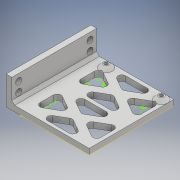
# Autodesk Inventor part: OpenMV
Saved by Autodesk Inventor 2018 (Build 220112000, 112)
## iProperties
Created: 2018-09-23
Part Number: OpenMV
Material: 一般
Document SubType Name: Modeling
Designer: shun2
Density: 1 g/cm^3
Appearance: 既定
Author: shun2
Autodesk Inventor part; units mm, degrees
ref_plane "YZ Plane" through (0, 0, 0) normal (1, 0, 0) x (0, 1, 0)
ref_plane "XZ Plane" through (0, 0, 0) normal (0, 1, 0) x (-1, 0, 0)
ref_plane "XY Plane" through (0, 0, 0) normal (0, 0, 1) x (1, 0, 0)
sketch "スケッチ2" plane through (0, 0, 0) normal (0, 0, 1) x (1, 0, 0)
  line L0 (0, 44.45) -> (0, 0)
  line L1 (0, 0) -> (35.56, 0)
  line L2 (35.56, 0) -> (35.56, 44.45)
  line L3 (35.56, 44.45) -> (0, 44.45)
  arc A0 (0.381, 41.1607) -> (0.381, 41.1353) centre (0.381, 41.148) ccw
  arc A1 (6.223, 41.1353) -> (6.223, 41.1607) centre (6.223, 41.148) ccw
  arc A2 (3.302, 38.227) -> (3.302, 44.069) centre (3.302, 41.148) ccw
  arc A3 (3.302, 44.069) -> (3.302, 38.227) centre (3.302, 41.148) ccw
  arc A4 (3.302, 39.648) -> (3.302, 42.648) centre (3.302, 41.148) ccw
  arc A5 (3.302, 42.648) -> (3.302, 39.648) centre (3.302, 41.148) ccw
  line L4 (35.179, 41.148) -> (34.925, 41.148)
  arc A6 (34.925, 41.1607) -> (34.925, 41.1353) centre (34.925, 41.148) ccw
  arc A7 (35.179, 41.1353) -> (35.179, 41.1607) centre (35.179, 41.148) ccw
  arc A8 (29.337, 41.1607) -> (29.337, 41.1353) centre (29.337, 41.148) ccw
  arc A9 (32.258, 38.227) -> (32.258, 44.069) centre (32.258, 41.148) ccw
  arc A10 (32.258, 44.069) -> (32.258, 38.227) centre (32.258, 41.148) ccw
  arc A11 (32.258, 39.648) -> (32.258, 42.648) centre (32.258, 41.148) ccw
  arc A12 (32.258, 42.648) -> (32.258, 39.648) centre (32.258, 41.148) ccw
  line L5 (35.179, 4.699) -> (35.179, 3.429)
  arc A13 (35.1409, 3.429) -> (35.2171, 3.429) centre (35.179, 3.429) ccw
  arc A14 (35.2171, 4.699) -> (35.1409, 4.699) centre (35.179, 4.699) ccw
  line L6 (35.179, 3.429) -> (34.544, 2.794)
  arc A15 (34.5171, 2.8209) -> (34.5709, 2.7671) centre (34.544, 2.794) ccw
  arc A16 (35.2059, 3.4021) -> (35.1521, 3.4559) centre (35.179, 3.429) ccw
  arc A17 (33.274, 2.8321) -> (33.274, 2.7559) centre (33.274, 2.794) ccw
  arc A18 (34.544, 2.7559) -> (34.544, 2.8321) centre (34.544, 2.794) ccw
  line L7 (33.274, 2.794) -> (32.639, 3.429)
  arc A19 (32.6659, 3.4559) -> (32.6121, 3.4021) centre (32.639, 3.429) ccw
  arc A20 (33.2471, 2.7671) -> (33.3009, 2.8209) centre (33.274, 2.794) ccw
  line L8 (34.544, 7.874) -> (35.179, 7.239)
  arc A21 (35.1521, 7.2121) -> (35.2059, 7.2659) centre (35.179, 7.239) ccw
  arc A22 (34.5709, 7.9009) -> (34.5171, 7.8471) centre (34.544, 7.874) ccw
  line L9 (35.179, 7.239) -> (35.179, 5.969)
  arc A23 (35.1409, 5.969) -> (35.2171, 5.969) centre (35.179, 5.969) ccw
  arc A24 (35.2171, 7.239) -> (35.1409, 7.239) centre (35.179, 7.239) ccw
  line L10 (35.179, 5.969) -> (34.544, 5.334)
  arc A25 (34.5171, 5.3609) -> (34.5709, 5.3071) centre (34.544, 5.334) ccw
  arc A26 (35.2059, 5.9421) -> (35.1521, 5.9959) centre (35.179, 5.969) ccw
  arc A27 (33.274, 5.3721) -> (33.274, 5.2959) centre (33.274, 5.334) ccw
  arc A28 (34.544, 5.2959) -> (34.544, 5.3721) centre (34.544, 5.334) ccw
  line L11 (33.274, 5.334) -> (32.639, 5.969)
  arc A29 (32.6659, 5.9959) -> (32.6121, 5.9421) centre (32.639, 5.969) ccw
  arc A30 (33.2471, 5.3071) -> (33.3009, 5.3609) centre (33.274, 5.334) ccw
  line L12 (32.639, 5.969) -> (32.639, 7.239)
  arc A31 (32.6771, 7.239) -> (32.6009, 7.239) centre (32.639, 7.239) ccw
  arc A32 (32.6009, 5.969) -> (32.6771, 5.969) centre (32.639, 5.969) ccw
  line L13 (32.639, 7.239) -> (33.274, 7.874)
  arc A33 (33.3009, 7.8471) -> (33.2471, 7.9009) centre (33.274, 7.874) ccw
  arc A34 (32.6121, 7.2659) -> (32.6659, 7.2121) centre (32.639, 7.239) ccw
  line L14 (35.179, 4.699) -> (34.544, 5.334)
  arc A35 (34.5709, 5.3609) -> (34.5171, 5.3071) centre (34.544, 5.334) ccw
  arc A36 (35.1521, 4.6721) -> (35.2059, 4.7259) centre (35.179, 4.699) ccw
  line L15 (33.274, 5.334) -> (32.639, 4.699)
  arc A37 (32.6121, 4.7259) -> (32.6659, 4.6721) centre (32.639, 4.699) ccw
  arc A38 (33.3009, 5.3071) -> (33.2471, 5.3609) centre (33.274, 5.334) ccw
  line L16 (32.639, 3.429) -> (32.639, 4.699)
  arc A39 (32.6771, 4.699) -> (32.6009, 4.699) centre (32.639, 4.699) ccw
  arc A40 (32.6009, 3.429) -> (32.6771, 3.429) centre (32.639, 3.429) ccw
  line L17 (35.179, 12.319) -> (35.179, 11.049)
  arc A41 (35.1409, 11.049) -> (35.2171, 11.049) centre (35.179, 11.049) ccw
  arc A42 (35.2171, 12.319) -> (35.1409, 12.319) centre (35.179, 12.319) ccw
  line L18 (35.179, 11.049) -> (34.544, 10.414)
  arc A43 (34.5171, 10.4409) -> (34.5709, 10.3871) centre (34.544, 10.414) ccw
  arc A44 (35.2059, 11.0221) -> (35.1521, 11.0759) centre (35.179, 11.049) ccw
  arc A45 (33.274, 10.4521) -> (33.274, 10.3759) centre (33.274, 10.414) ccw
  arc A46 (34.544, 10.3759) -> (34.544, 10.4521) centre (34.544, 10.414) ccw
  line L19 (33.274, 10.414) -> (32.639, 11.049)
  arc A47 (32.6659, 11.0759) -> (32.6121, 11.0221) centre (32.639, 11.049) ccw
  arc A48 (33.2471, 10.3871) -> (33.3009, 10.4409) centre (33.274, 10.414) ccw
  line L20 (34.544, 10.414) -> (35.179, 9.779)
  arc A49 (35.1521, 9.7521) -> (35.2059, 9.8059) centre (35.179, 9.779) ccw
  arc A50 (34.5709, 10.4409) -> (34.5171, 10.3871) centre (34.544, 10.414) ccw
  line L21 (35.179, 9.779) -> (35.179, 8.509)
  arc A51 (35.1409, 8.509) -> (35.2171, 8.509) centre (35.179, 8.509) ccw
  arc A52 (35.2171, 9.779) -> (35.1409, 9.779) centre (35.179, 9.779) ccw
  line L22 (35.179, 8.509) -> (34.544, 7.874)
  arc A53 (34.5171, 7.9009) -> (34.5709, 7.8471) centre (34.544, 7.874) ccw
  arc A54 (35.2059, 8.4821) -> (35.1521, 8.5359) centre (35.179, 8.509) ccw
  arc A55 (33.274, 7.9121) -> (33.274, 7.8359) centre (33.274, 7.874) ccw
  arc A56 (34.544, 7.8359) -> (34.544, 7.9121) centre (34.544, 7.874) ccw
  line L23 (33.274, 7.874) -> (32.639, 8.509)
  arc A57 (32.6659, 8.5359) -> (32.6121, 8.4821) centre (32.639, 8.509) ccw
  arc A58 (33.2471, 7.8471) -> (33.3009, 7.9009) centre (33.274, 7.874) ccw
  line L24 (32.639, 8.509) -> (32.639, 9.779)
  arc A59 (32.6771, 9.779) -> (32.6009, 9.779) centre (32.639, 9.779) ccw
  arc A60 (32.6009, 8.509) -> (32.6771, 8.509) centre (32.639, 8.509) ccw
  line L25 (32.639, 9.779) -> (33.274, 10.414)
  arc A61 (33.3009, 10.3871) -> (33.2471, 10.4409) centre (33.274, 10.414) ccw
  arc A62 (32.6121, 9.8059) -> (32.6659, 9.7521) centre (32.639, 9.779) ccw
  line L26 (34.544, 15.494) -> (35.179, 14.859)
  arc A63 (35.1521, 14.8321) -> (35.2059, 14.8859) centre (35.179, 14.859) ccw
  arc A64 (34.5709, 15.5209) -> (34.5171, 15.4671) centre (34.544, 15.494) ccw
  line L27 (35.179, 14.859) -> (35.179, 13.589)
  arc A65 (35.1409, 13.589) -> (35.2171, 13.589) centre (35.179, 13.589) ccw
  arc A66 (35.2171, 14.859) -> (35.1409, 14.859) centre (35.179, 14.859) ccw
  line L28 (35.179, 13.589) -> (34.544, 12.954)
  arc A67 (34.5171, 12.9809) -> (34.5709, 12.9271) centre (34.544, 12.954) ccw
  arc A68 (35.2059, 13.5621) -> (35.1521, 13.6159) centre (35.179, 13.589) ccw
  arc A69 (33.274, 12.9921) -> (33.274, 12.9159) centre (33.274, 12.954) ccw
  arc A70 (34.544, 12.9159) -> (34.544, 12.9921) centre (34.544, 12.954) ccw
  line L29 (33.274, 12.954) -> (32.639, 13.589)
  arc A71 (32.6659, 13.6159) -> (32.6121, 13.5621) centre (32.639, 13.589) ccw
  arc A72 (33.2471, 12.9271) -> (33.3009, 12.9809) centre (33.274, 12.954) ccw
  line L30 (32.639, 13.589) -> (32.639, 14.859)
  arc A73 (32.6771, 14.859) -> (32.6009, 14.859) centre (32.639, 14.859) ccw
  arc A74 (32.6009, 13.589) -> (32.6771, 13.589) centre (32.639, 13.589) ccw
  line L31 (32.639, 14.859) -> (33.274, 15.494)
  arc A75 (33.3009, 15.4671) -> (33.2471, 15.5209) centre (33.274, 15.494) ccw
  arc A76 (32.6121, 14.8859) -> (32.6659, 14.8321) centre (32.639, 14.859) ccw
  line L32 (35.179, 12.319) -> (34.544, 12.954)
  arc A77 (34.5709, 12.9809) -> (34.5171, 12.9271) centre (34.544, 12.954) ccw
  arc A78 (35.1521, 12.2921) -> (35.2059, 12.3459) centre (35.179, 12.319) ccw
  line L33 (33.274, 12.954) -> (32.639, 12.319)
  arc A79 (32.6121, 12.3459) -> (32.6659, 12.2921) centre (32.639, 12.319) ccw
  arc A80 (33.3009, 12.9271) -> (33.2471, 12.9809) centre (33.274, 12.954) ccw
  line L34 (32.639, 11.049) -> (32.639, 12.319)
  arc A81 (32.6771, 12.319) -> (32.6009, 12.319) centre (32.639, 12.319) ccw
  arc A82 (32.6009, 11.049) -> (32.6771, 11.049) centre (32.639, 11.049) ccw
  line L35 (35.179, 19.939) -> (35.179, 18.669)
  arc A83 (35.1409, 18.669) -> (35.2171, 18.669) centre (35.179, 18.669) ccw
  arc A84 (35.2171, 19.939) -> (35.1409, 19.939) centre (35.179, 19.939) ccw
  line L36 (35.179, 18.669) -> (34.544, 18.034)
  arc A85 (34.5171, 18.0609) -> (34.5709, 18.0071) centre (34.544, 18.034) ccw
  arc A86 (35.2059, 18.6421) -> (35.1521, 18.6959) centre (35.179, 18.669) ccw
  arc A87 (33.274, 18.0721) -> (33.274, 17.9959) centre (33.274, 18.034) ccw
  arc A88 (34.544, 17.9959) -> (34.544, 18.0721) centre (34.544, 18.034) ccw
  line L37 (33.274, 18.034) -> (32.639, 18.669)
  arc A89 (32.6659, 18.6959) -> (32.6121, 18.6421) centre (32.639, 18.669) ccw
  arc A90 (33.2471, 18.0071) -> (33.3009, 18.0609) centre (33.274, 18.034) ccw
  line L38 (34.544, 18.034) -> (35.179, 17.399)
  arc A91 (35.1521, 17.3721) -> (35.2059, 17.4259) centre (35.179, 17.399) ccw
  arc A92 (34.5709, 18.0609) -> (34.5171, 18.0071) centre (34.544, 18.034) ccw
  line L39 (35.179, 17.399) -> (35.179, 16.129)
  arc A93 (35.1409, 16.129) -> (35.2171, 16.129) centre (35.179, 16.129) ccw
  arc A94 (35.2171, 17.399) -> (35.1409, 17.399) centre (35.179, 17.399) ccw
  line L40 (35.179, 16.129) -> (34.544, 15.494)
  arc A95 (34.5171, 15.5209) -> (34.5709, 15.4671) centre (34.544, 15.494) ccw
  arc A96 (35.2059, 16.1021) -> (35.1521, 16.1559) centre (35.179, 16.129) ccw
  arc A97 (33.274, 15.5321) -> (33.274, 15.4559) centre (33.274, 15.494) ccw
  arc A98 (34.544, 15.4559) -> (34.544, 15.5321) centre (34.544, 15.494) ccw
  line L41 (33.274, 15.494) -> (32.639, 16.129)
  arc A99 (32.6659, 16.1559) -> (32.6121, 16.1021) centre (32.639, 16.129) ccw
  arc A100 (33.2471, 15.4671) -> (33.3009, 15.5209) centre (33.274, 15.494) ccw
  line L42 (32.639, 16.129) -> (32.639, 17.399)
  arc A101 (32.6771, 17.399) -> (32.6009, 17.399) centre (32.639, 17.399) ccw
  arc A102 (32.6009, 16.129) -> (32.6771, 16.129) centre (32.639, 16.129) ccw
  line L43 (32.639, 17.399) -> (33.274, 18.034)
  arc A103 (33.3009, 18.0071) -> (33.2471, 18.0609) centre (33.274, 18.034) ccw
  arc A104 (32.6121, 17.4259) -> (32.6659, 17.3721) centre (32.639, 17.399) ccw
  line L44 (34.544, 20.574) -> (33.274, 20.574)
  arc A105 (33.274, 20.6121) -> (33.274, 20.5359) centre (33.274, 20.574) ccw
  arc A106 (34.544, 20.5359) -> (34.544, 20.6121) centre (34.544, 20.574) ccw
  line L45 (35.179, 19.939) -> (34.544, 20.574)
  arc A107 (34.5709, 20.6009) -> (34.5171, 20.5471) centre (34.544, 20.574) ccw
  arc A108 (35.1521, 19.9121) -> (35.2059, 19.9659) centre (35.179, 19.939) ccw
  line L46 (33.274, 20.574) -> (32.639, 19.939)
  arc A109 (32.6121, 19.9659) -> (32.6659, 19.9121) centre (32.639, 19.939) ccw
  arc A110 (33.3009, 20.5471) -> (33.2471, 20.6009) centre (33.274, 20.574) ccw
  line L47 (32.639, 18.669) -> (32.639, 19.939)
  arc A111 (32.6771, 19.939) -> (32.6009, 19.939) centre (32.639, 19.939) ccw
  arc A112 (32.6009, 18.669) -> (32.6771, 18.669) centre (32.639, 18.669) ccw
  line L48 (35.179, 2.159) -> (35.179, 0.889)
  arc A113 (35.1409, 0.889) -> (35.2171, 0.889) centre (35.179, 0.889) ccw
  arc A114 (35.2171, 2.159) -> (35.1409, 2.159) centre (35.179, 2.159) ccw
  line L49 (35.179, 0.889) -> (34.544, 0.254)
  arc A115 (34.5171, 0.2809) -> (34.5709, 0.2271) centre (34.544, 0.254) ccw
  arc A116 (35.2059, 0.8621) -> (35.1521, 0.9159) centre (35.179, 0.889) ccw
  line L50 (34.544, 0.254) -> (33.274, 0.254)
  arc A117 (33.274, 0.2921) -> (33.274, 0.2159) centre (33.274, 0.254) ccw
  arc A118 (34.544, 0.2159) -> (34.544, 0.2921) centre (34.544, 0.254) ccw
  line L51 (33.274, 0.254) -> (32.639, 0.889)
  arc A119 (32.6659, 0.9159) -> (32.6121, 0.8621) centre (32.639, 0.889) ccw
  arc A120 (33.2471, 0.2271) -> (33.3009, 0.2809) centre (33.274, 0.254) ccw
  line L52 (35.179, 2.159) -> (34.544, 2.794)
  arc A121 (34.5709, 2.8209) -> (34.5171, 2.7671) centre (34.544, 2.794) ccw
  arc A122 (35.1521, 2.1321) -> (35.2059, 2.1859) centre (35.179, 2.159) ccw
  line L53 (33.274, 2.794) -> (32.639, 2.159)
  arc A123 (32.6121, 2.1859) -> (32.6659, 2.1321) centre (32.639, 2.159) ccw
  arc A124 (33.3009, 2.7671) -> (33.2471, 2.8209) centre (33.274, 2.794) ccw
  line L54 (32.639, 0.889) -> (32.639, 2.159)
  arc A125 (32.6771, 2.159) -> (32.6009, 2.159) centre (32.639, 2.159) ccw
  arc A126 (32.6009, 0.889) -> (32.6771, 0.889) centre (32.639, 0.889) ccw
  line L55 (2.921, 4.699) -> (2.921, 3.429)
  arc A127 (2.8829, 3.429) -> (2.9591, 3.429) centre (2.921, 3.429) ccw
  arc A128 (2.9591, 4.699) -> (2.8829, 4.699) centre (2.921, 4.699) ccw
  line L56 (2.921, 3.429) -> (2.286, 2.794)
  arc A129 (2.2591, 2.8209) -> (2.3129, 2.7671) centre (2.286, 2.794) ccw
  arc A130 (2.9479, 3.4021) -> (2.8941, 3.4559) centre (2.921, 3.429) ccw
  arc A131 (1.016, 2.8321) -> (1.016, 2.7559) centre (1.016, 2.794) ccw
  arc A132 (2.286, 2.7559) -> (2.286, 2.8321) centre (2.286, 2.794) ccw
  line L57 (1.016, 2.794) -> (0.381, 3.429)
  arc A133 (0.4079, 3.4559) -> (0.3541, 3.4021) centre (0.381, 3.429) ccw
  arc A134 (0.9891, 2.7671) -> (1.0429, 2.8209) centre (1.016, 2.794) ccw
  line L58 (2.286, 7.874) -> (2.921, 7.239)
  arc A135 (2.8941, 7.2121) -> (2.9479, 7.2659) centre (2.921, 7.239) ccw
  arc A136 (2.3129, 7.9009) -> (2.2591, 7.8471) centre (2.286, 7.874) ccw
  line L59 (2.921, 7.239) -> (2.921, 5.969)
  arc A137 (2.8829, 5.969) -> (2.9591, 5.969) centre (2.921, 5.969) ccw
  arc A138 (2.9591, 7.239) -> (2.8829, 7.239) centre (2.921, 7.239) ccw
  line L60 (2.921, 5.969) -> (2.286, 5.334)
  arc A139 (2.2591, 5.3609) -> (2.3129, 5.3071) centre (2.286, 5.334) ccw
  arc A140 (2.9479, 5.9421) -> (2.8941, 5.9959) centre (2.921, 5.969) ccw
  arc A141 (1.016, 5.3721) -> (1.016, 5.2959) centre (1.016, 5.334) ccw
  arc A142 (2.286, 5.2959) -> (2.286, 5.3721) centre (2.286, 5.334) ccw
  line L61 (1.016, 5.334) -> (0.381, 5.969)
  arc A143 (0.4079, 5.9959) -> (0.3541, 5.9421) centre (0.381, 5.969) ccw
  arc A144 (0.9891, 5.3071) -> (1.0429, 5.3609) centre (1.016, 5.334) ccw
  line L62 (0.381, 5.969) -> (0.381, 7.239)
  arc A145 (0.4191, 7.239) -> (0.3429, 7.239) centre (0.381, 7.239) ccw
  arc A146 (0.3429, 5.969) -> (0.4191, 5.969) centre (0.381, 5.969) ccw
  line L63 (0.381, 7.239) -> (1.016, 7.874)
  arc A147 (1.0429, 7.8471) -> (0.9891, 7.9009) centre (1.016, 7.874) ccw
  arc A148 (0.3541, 7.2659) -> (0.4079, 7.2121) centre (0.381, 7.239) ccw
  line L64 (2.921, 4.699) -> (2.286, 5.334)
  arc A149 (2.3129, 5.3609) -> (2.2591, 5.3071) centre (2.286, 5.334) ccw
  arc A150 (2.8941, 4.6721) -> (2.9479, 4.7259) centre (2.921, 4.699) ccw
  line L65 (1.016, 5.334) -> (0.381, 4.699)
  arc A151 (0.3541, 4.7259) -> (0.4079, 4.6721) centre (0.381, 4.699) ccw
  arc A152 (1.0429, 5.3071) -> (0.9891, 5.3609) centre (1.016, 5.334) ccw
  line L66 (0.381, 3.429) -> (0.381, 4.699)
  arc A153 (0.4191, 4.699) -> (0.3429, 4.699) centre (0.381, 4.699) ccw
  arc A154 (0.3429, 3.429) -> (0.4191, 3.429) centre (0.381, 3.429) ccw
  line L67 (2.921, 12.319) -> (2.921, 11.049)
  arc A155 (2.8829, 11.049) -> (2.9591, 11.049) centre (2.921, 11.049) ccw
  arc A156 (2.9591, 12.319) -> (2.8829, 12.319) centre (2.921, 12.319) ccw
  line L68 (2.921, 11.049) -> (2.286, 10.414)
  arc A157 (2.2591, 10.4409) -> (2.3129, 10.3871) centre (2.286, 10.414) ccw
  arc A158 (2.9479, 11.0221) -> (2.8941, 11.0759) centre (2.921, 11.049) ccw
  arc A159 (1.016, 10.4521) -> (1.016, 10.3759) centre (1.016, 10.414) ccw
  arc A160 (2.286, 10.3759) -> (2.286, 10.4521) centre (2.286, 10.414) ccw
  line L69 (1.016, 10.414) -> (0.381, 11.049)
  arc A161 (0.4079, 11.0759) -> (0.3541, 11.0221) centre (0.381, 11.049) ccw
  arc A162 (0.9891, 10.3871) -> (1.0429, 10.4409) centre (1.016, 10.414) ccw
  line L70 (2.286, 10.414) -> (2.921, 9.779)
  arc A163 (2.8941, 9.7521) -> (2.9479, 9.8059) centre (2.921, 9.779) ccw
  arc A164 (2.3129, 10.4409) -> (2.2591, 10.3871) centre (2.286, 10.414) ccw
  line L71 (2.921, 9.779) -> (2.921, 8.509)
  arc A165 (2.8829, 8.509) -> (2.9591, 8.509) centre (2.921, 8.509) ccw
  arc A166 (2.9591, 9.779) -> (2.8829, 9.779) centre (2.921, 9.779) ccw
  line L72 (2.921, 8.509) -> (2.286, 7.874)
  arc A167 (2.2591, 7.9009) -> (2.3129, 7.8471) centre (2.286, 7.874) ccw
  arc A168 (2.9479, 8.4821) -> (2.8941, 8.5359) centre (2.921, 8.509) ccw
  arc A169 (1.016, 7.9121) -> (1.016, 7.8359) centre (1.016, 7.874) ccw
  arc A170 (2.286, 7.8359) -> (2.286, 7.9121) centre (2.286, 7.874) ccw
  line L73 (1.016, 7.874) -> (0.381, 8.509)
  arc A171 (0.4079, 8.5359) -> (0.3541, 8.4821) centre (0.381, 8.509) ccw
  arc A172 (0.9891, 7.8471) -> (1.0429, 7.9009) centre (1.016, 7.874) ccw
  line L74 (0.381, 8.509) -> (0.381, 9.779)
  arc A173 (0.4191, 9.779) -> (0.3429, 9.779) centre (0.381, 9.779) ccw
  arc A174 (0.3429, 8.509) -> (0.4191, 8.509) centre (0.381, 8.509) ccw
  line L75 (0.381, 9.779) -> (1.016, 10.414)
  arc A175 (1.0429, 10.3871) -> (0.9891, 10.4409) centre (1.016, 10.414) ccw
  arc A176 (0.3541, 9.8059) -> (0.4079, 9.7521) centre (0.381, 9.779) ccw
  line L76 (2.286, 15.494) -> (2.921, 14.859)
  arc A177 (2.8941, 14.8321) -> (2.9479, 14.8859) centre (2.921, 14.859) ccw
  arc A178 (2.3129, 15.5209) -> (2.2591, 15.4671) centre (2.286, 15.494) ccw
  line L77 (2.921, 14.859) -> (2.921, 13.589)
  arc A179 (2.8829, 13.589) -> (2.9591, 13.589) centre (2.921, 13.589) ccw
  arc A180 (2.9591, 14.859) -> (2.8829, 14.859) centre (2.921, 14.859) ccw
  line L78 (2.921, 13.589) -> (2.286, 12.954)
  arc A181 (2.2591, 12.9809) -> (2.3129, 12.9271) centre (2.286, 12.954) ccw
  arc A182 (2.9479, 13.5621) -> (2.8941, 13.6159) centre (2.921, 13.589) ccw
  arc A183 (1.016, 12.9921) -> (1.016, 12.9159) centre (1.016, 12.954) ccw
  arc A184 (2.286, 12.9159) -> (2.286, 12.9921) centre (2.286, 12.954) ccw
  line L79 (1.016, 12.954) -> (0.381, 13.589)
  arc A185 (0.4079, 13.6159) -> (0.3541, 13.5621) centre (0.381, 13.589) ccw
  arc A186 (0.9891, 12.9271) -> (1.0429, 12.9809) centre (1.016, 12.954) ccw
  line L80 (0.381, 13.589) -> (0.381, 14.859)
  arc A187 (0.4191, 14.859) -> (0.3429, 14.859) centre (0.381, 14.859) ccw
  arc A188 (0.3429, 13.589) -> (0.4191, 13.589) centre (0.381, 13.589) ccw
  line L81 (0.381, 14.859) -> (1.016, 15.494)
  arc A189 (1.0429, 15.4671) -> (0.9891, 15.5209) centre (1.016, 15.494) ccw
  arc A190 (0.3541, 14.8859) -> (0.4079, 14.8321) centre (0.381, 14.859) ccw
  line L82 (2.921, 12.319) -> (2.286, 12.954)
  arc A191 (2.3129, 12.9809) -> (2.2591, 12.9271) centre (2.286, 12.954) ccw
  arc A192 (2.8941, 12.2921) -> (2.9479, 12.3459) centre (2.921, 12.319) ccw
  line L83 (1.016, 12.954) -> (0.381, 12.319)
  arc A193 (0.3541, 12.3459) -> (0.4079, 12.2921) centre (0.381, 12.319) ccw
  arc A194 (1.0429, 12.9271) -> (0.9891, 12.9809) centre (1.016, 12.954) ccw
  line L84 (0.381, 11.049) -> (0.381, 12.319)
  arc A195 (0.4191, 12.319) -> (0.3429, 12.319) centre (0.381, 12.319) ccw
  arc A196 (0.3429, 11.049) -> (0.4191, 11.049) centre (0.381, 11.049) ccw
  line L85 (2.921, 19.939) -> (2.921, 18.669)
  arc A197 (2.8829, 18.669) -> (2.9591, 18.669) centre (2.921, 18.669) ccw
  arc A198 (2.9591, 19.939) -> (2.8829, 19.939) centre (2.921, 19.939) ccw
  line L86 (2.921, 18.669) -> (2.286, 18.034)
  arc A199 (2.2591, 18.0609) -> (2.3129, 18.0071) centre (2.286, 18.034) ccw
  arc A200 (2.9479, 18.6421) -> (2.8941, 18.6959) centre (2.921, 18.669) ccw
  arc A201 (1.016, 18.0721) -> (1.016, 17.9959) centre (1.016, 18.034) ccw
  arc A202 (2.286, 17.9959) -> (2.286, 18.0721) centre (2.286, 18.034) ccw
  line L87 (1.016, 18.034) -> (0.381, 18.669)
  arc A203 (0.4079, 18.6959) -> (0.3541, 18.6421) centre (0.381, 18.669) ccw
  arc A204 (0.9891, 18.0071) -> (1.0429, 18.0609) centre (1.016, 18.034) ccw
  line L88 (2.286, 18.034) -> (2.921, 17.399)
  arc A205 (2.8941, 17.3721) -> (2.9479, 17.4259) centre (2.921, 17.399) ccw
  arc A206 (2.3129, 18.0609) -> (2.2591, 18.0071) centre (2.286, 18.034) ccw
  line L89 (2.921, 17.399) -> (2.921, 16.129)
  arc A207 (2.8829, 16.129) -> (2.9591, 16.129) centre (2.921, 16.129) ccw
  arc A208 (2.9591, 17.399) -> (2.8829, 17.399) centre (2.921, 17.399) ccw
  line L90 (2.921, 16.129) -> (2.286, 15.494)
  arc A209 (2.2591, 15.5209) -> (2.3129, 15.4671) centre (2.286, 15.494) ccw
  arc A210 (2.9479, 16.1021) -> (2.8941, 16.1559) centre (2.921, 16.129) ccw
  arc A211 (1.016, 15.5321) -> (1.016, 15.4559) centre (1.016, 15.494) ccw
  arc A212 (2.286, 15.4559) -> (2.286, 15.5321) centre (2.286, 15.494) ccw
  line L91 (1.016, 15.494) -> (0.381, 16.129)
  arc A213 (0.4079, 16.1559) -> (0.3541, 16.1021) centre (0.381, 16.129) ccw
  arc A214 (0.9891, 15.4671) -> (1.0429, 15.5209) centre (1.016, 15.494) ccw
  line L92 (0.381, 16.129) -> (0.381, 17.399)
  arc A215 (0.4191, 17.399) -> (0.3429, 17.399) centre (0.381, 17.399) ccw
  arc A216 (0.3429, 16.129) -> (0.4191, 16.129) centre (0.381, 16.129) ccw
  line L93 (0.381, 17.399) -> (1.016, 18.034)
  arc A217 (1.0429, 18.0071) -> (0.9891, 18.0609) centre (1.016, 18.034) ccw
  arc A218 (0.3541, 17.4259) -> (0.4079, 17.3721) centre (0.381, 17.399) ccw
  line L94 (2.286, 20.574) -> (1.016, 20.574)
  arc A219 (1.016, 20.6121) -> (1.016, 20.5359) centre (1.016, 20.574) ccw
  arc A220 (2.286, 20.5359) -> (2.286, 20.6121) centre (2.286, 20.574) ccw
  line L95 (2.921, 19.939) -> (2.286, 20.574)
  arc A221 (2.3129, 20.6009) -> (2.2591, 20.5471) centre (2.286, 20.574) ccw
  arc A222 (2.8941, 19.9121) -> (2.9479, 19.9659) centre (2.921, 19.939) ccw
  line L96 (1.016, 20.574) -> (0.381, 19.939)
  arc A223 (0.3541, 19.9659) -> (0.4079, 19.9121) centre (0.381, 19.939) ccw
  arc A224 (1.0429, 20.5471) -> (0.9891, 20.6009) centre (1.016, 20.574) ccw
  line L97 (0.381, 18.669) -> (0.381, 19.939)
  arc A225 (0.4191, 19.939) -> (0.3429, 19.939) centre (0.381, 19.939) ccw
  arc A226 (0.3429, 18.669) -> (0.4191, 18.669) centre (0.381, 18.669) ccw
  line L98 (2.921, 2.159) -> (2.921, 0.889)
  arc A227 (2.8829, 0.889) -> (2.9591, 0.889) centre (2.921, 0.889) ccw
  arc A228 (2.9591, 2.159) -> (2.8829, 2.159) centre (2.921, 2.159) ccw
  line L99 (2.921, 0.889) -> (2.286, 0.254)
  arc A229 (2.2591, 0.2809) -> (2.3129, 0.2271) centre (2.286, 0.254) ccw
  arc A230 (2.9479, 0.8621) -> (2.8941, 0.9159) centre (2.921, 0.889) ccw
  line L100 (2.286, 0.254) -> (1.016, 0.254)
  arc A231 (1.016, 0.2921) -> (1.016, 0.2159) centre (1.016, 0.254) ccw
  arc A232 (2.286, 0.2159) -> (2.286, 0.2921) centre (2.286, 0.254) ccw
  line L101 (1.016, 0.254) -> (0.381, 0.889)
  arc A233 (0.4079, 0.9159) -> (0.3541, 0.8621) centre (0.381, 0.889) ccw
  arc A234 (0.9891, 0.2271) -> (1.0429, 0.2809) centre (1.016, 0.254) ccw
  line L102 (2.921, 2.159) -> (2.286, 2.794)
  arc A235 (2.3129, 2.8209) -> (2.2591, 2.7671) centre (2.286, 2.794) ccw
  arc A236 (2.8941, 2.1321) -> (2.9479, 2.1859) centre (2.921, 2.159) ccw
  line L103 (1.016, 2.794) -> (0.381, 2.159)
  arc A237 (0.3541, 2.1859) -> (0.4079, 2.1321) centre (0.381, 2.159) ccw
  arc A238 (1.0429, 2.7671) -> (0.9891, 2.8209) centre (1.016, 2.794) ccw
  line L104 (0.381, 0.889) -> (0.381, 2.159)
  arc A239 (0.4191, 2.159) -> (0.3429, 2.159) centre (0.381, 2.159) ccw
  arc A240 (0.3429, 0.889) -> (0.4191, 0.889) centre (0.381, 0.889) ccw
  line L105 (1.24, 31.399) -> (0.94, 31.399)
  arc A241 (0.94, 31.4498) -> (0.94, 31.3482) centre (0.94, 31.399) ccw
  arc A242 (1.24, 31.3482) -> (1.24, 31.4498) centre (1.24, 31.399) ccw
  line L106 (0.94, 31.399) -> (0.94, 28.799)
  arc A243 (0.8892, 28.799) -> (0.9908, 28.799) centre (0.94, 28.799) ccw
  arc A244 (0.9908, 31.399) -> (0.8892, 31.399) centre (0.94, 31.399) ccw
  line L107 (0.94, 28.799) -> (1.24, 28.799)
  arc A245 (1.24, 28.7482) -> (1.24, 28.8498) centre (1.24, 28.799) ccw
  arc A246 (0.94, 28.8498) -> (0.94, 28.7482) centre (0.94, 28.799) ccw
  line L108 (3.84, 31.399) -> (4.14, 31.399)
  arc A247 (4.14, 31.3482) -> (4.14, 31.4498) centre (4.14, 31.399) ccw
  arc A248 (3.84, 31.4498) -> (3.84, 31.3482) centre (3.84, 31.399) ccw
  line L109 (4.14, 31.399) -> (4.14, 28.799)
  arc A249 (4.0892, 28.799) -> (4.1908, 28.799) centre (4.14, 28.799) ccw
  arc A250 (4.1908, 31.399) -> (4.0892, 31.399) centre (4.14, 31.399) ccw
  line L110 (4.14, 28.799) -> (3.84, 28.799)
  arc A251 (3.84, 28.8498) -> (3.84, 28.7482) centre (3.84, 28.799) ccw
  arc A252 (4.14, 28.7482) -> (4.14, 28.8498) centre (4.14, 28.799) ccw
  line L111 (9.78, 28.068) -> (9.78, 34.091)
  arc A253 (9.8118, 34.091) -> (9.7483, 34.091) centre (9.78, 34.091) ccw
  arc A254 (9.7483, 28.068) -> (9.8118, 28.068) centre (9.78, 28.068) ccw
  line L112 (9.78, 34.091) -> (9.78, 38.045)
  arc A255 (9.8118, 38.045) -> (9.7483, 38.045) centre (9.78, 38.045) ccw
  arc A256 (9.7483, 34.091) -> (9.8118, 34.091) centre (9.78, 34.091) ccw
  line L113 (9.78, 38.045) -> (9.78, 44.068)
  arc A257 (9.8118, 44.068) -> (9.7483, 44.068) centre (9.78, 44.068) ccw
  arc A258 (9.7483, 38.045) -> (9.8118, 38.045) centre (9.78, 38.045) ccw
  line L114 (9.78, 44.068) -> (25.78, 44.068)
  arc A259 (25.78, 44.0363) -> (25.78, 44.0998) centre (25.78, 44.068) ccw
  arc A260 (9.78, 44.0998) -> (9.78, 44.0363) centre (9.78, 44.068) ccw
  line L115 (25.78, 44.068) -> (25.78, 38.045)
  arc A261 (25.7483, 38.045) -> (25.8117, 38.045) centre (25.78, 38.045) ccw
  arc A262 (25.8117, 44.068) -> (25.7483, 44.068) centre (25.78, 44.068) ccw
  line L116 (25.78, 38.045) -> (25.78, 34.091)
  arc A263 (25.7483, 34.091) -> (25.8117, 34.091) centre (25.78, 34.091) ccw
  arc A264 (25.8117, 38.045) -> (25.7483, 38.045) centre (25.78, 38.045) ccw
  line L117 (25.78, 34.091) -> (25.78, 28.068)
  arc A265 (25.7483, 28.068) -> (25.8117, 28.068) centre (25.78, 28.068) ccw
  arc A266 (25.8117, 34.091) -> (25.7483, 34.091) centre (25.78, 34.091) ccw
  line L118 (25.78, 28.068) -> (9.78, 28.068)
  arc A267 (9.78, 28.0998) -> (9.78, 28.0363) centre (9.78, 28.0681) ccw
  arc A268 (25.78, 28.0363) -> (25.78, 28.0998) centre (25.78, 28.0681) ccw
  arc A269 (9.78, 38.045) -> (9.78, 34.091) centre (7.803, 36.068) ccw
  arc A270 (9.7575, 38.0225) -> (9.8025, 38.0675) centre (9.78, 38.045) ccw
  arc A271 (9.8025, 34.0685) -> (9.7575, 34.1135) centre (9.78, 34.091) ccw
  arc A272 (25.78, 34.091) -> (25.78, 38.045) centre (27.757, 36.068) ccw
  arc A273 (25.8025, 34.1135) -> (25.7575, 34.0685) centre (25.78, 34.091) ccw
  arc A274 (25.7575, 38.0675) -> (25.8025, 38.0225) centre (25.78, 38.045) ccw
  line L119 (35.466, 20.943) -> (35.466, 32.943)
  arc A275 (35.4978, 32.943) -> (35.4342, 32.943) centre (35.466, 32.943) ccw
  arc A276 (35.4342, 20.943) -> (35.4978, 20.943) centre (35.466, 20.943) ccw
  line L120 (35.466, 32.943) -> (29.866, 32.943)
  arc A277 (29.866, 32.9748) -> (29.866, 32.9113) centre (29.866, 32.943) ccw
  arc A278 (35.466, 32.9113) -> (35.466, 32.9748) centre (35.466, 32.943) ccw
  line L121 (29.866, 32.943) -> (29.866, 20.943)
  arc A279 (29.8977, 32.943) -> (29.8343, 32.943) centre (29.866, 32.943) ccw
  line L122 (29.866, 20.943) -> (35.466, 20.943)
  arc A280 (35.466, 20.9113) -> (35.466, 20.9748) centre (35.466, 20.943) ccw
  line L123 (22.09, 0.0025) -> (31.25, 0.0025)
  arc A281 (31.25, -0.0293) -> (31.25, 0.0343) centre (31.25, 0.0025) ccw
  arc A282 (22.09, 0.0343) -> (22.09, -0.0293) centre (22.09, 0.0025) ccw
  line L124 (22.09, 0.0025) -> (22.09, 5.1575)
  arc A283 (22.1217, 5.1575) -> (22.0583, 5.1575) centre (22.09, 5.1575) ccw
  arc A284 (22.0583, 0.0025) -> (22.1217, 0.0025) centre (22.09, 0.0025) ccw
  line L125 (22.09, 5.1575) -> (31.25, 5.1575)
  arc A285 (31.25, 5.1258) -> (31.25, 5.1893) centre (31.25, 5.1576) ccw
  arc A286 (22.09, 5.1893) -> (22.09, 5.1258) centre (22.09, 5.1576) ccw
  line L126 (31.25, 5.1575) -> (31.25, 0.0025)
  arc A287 (31.2183, 0.0025) -> (31.2817, 0.0025) centre (31.25, 0.0025) ccw
  arc A288 (31.2817, 5.1575) -> (31.2183, 5.1575) centre (31.25, 5.1575) ccw
  arc A289 (7.874, 42.803) -> (7.874, 43.303) centre (7.874, 43.053) ccw
  arc A290 (7.874, 43.303) -> (7.874, 42.803) centre (7.874, 43.053) ccw
  arc A291 (7.874, 42.803) -> (7.874, 43.303) centre (7.874, 43.053) ccw
  arc A292 (7.874, 43.303) -> (7.874, 42.803) centre (7.874, 43.053) ccw
  arc A293 (4.6355, 41.148) -> (1.9685, 41.148) centre (3.302, 41.148) ccw
  arc A294 (1.9685, 41.148) -> (4.6355, 41.148) centre (3.302, 41.148) ccw
  arc A295 (4.256, 41.148) -> (2.348, 41.148) centre (3.302, 41.148) ccw
  arc A296 (2.348, 41.148) -> (4.256, 41.148) centre (3.302, 41.148) ccw
  arc A297 (4.256, 41.148) -> (2.348, 41.148) centre (3.302, 41.148) ccw
  arc A298 (2.348, 41.148) -> (4.256, 41.148) centre (3.302, 41.148) ccw
  arc A299 (4.6355, 41.148) -> (1.9685, 41.148) centre (3.302, 41.148) ccw
  arc A300 (1.9685, 41.148) -> (4.6355, 41.148) centre (3.302, 41.148) ccw
  arc A301 (30.9245, 41.148) -> (33.5915, 41.148) centre (32.258, 41.148) ccw
  arc A302 (33.5915, 41.148) -> (30.9245, 41.148) centre (32.258, 41.148) ccw
  arc A303 (31.304, 41.148) -> (33.212, 41.148) centre (32.258, 41.148) ccw
  arc A304 (33.212, 41.148) -> (31.304, 41.148) centre (32.258, 41.148) ccw
  arc A305 (31.304, 41.148) -> (33.212, 41.148) centre (32.258, 41.148) ccw
  arc A306 (33.212, 41.148) -> (31.304, 41.148) centre (32.258, 41.148) ccw
  arc A307 (30.9245, 41.148) -> (33.5915, 41.148) centre (32.258, 41.148) ccw
  arc A308 (33.5915, 41.148) -> (30.9245, 41.148) centre (32.258, 41.148) ccw
  line L127 (2.74, 31.099) -> (3.74, 31.099)
  line L128 (3.74, 31.099) -> (3.74, 32.099)
  line L129 (3.74, 32.099) -> (2.74, 32.099)
  line L130 (2.74, 32.099) -> (2.74, 31.099)
  line L131 (2.74, 28.099) -> (3.74, 28.099)
  line L132 (3.74, 28.099) -> (3.74, 29.099)
  line L133 (3.74, 29.099) -> (2.74, 29.099)
  line L134 (2.74, 29.099) -> (2.74, 28.099)
  line L135 (1.34, 28.099) -> (2.34, 28.099)
  line L136 (2.34, 28.099) -> (2.34, 29.099)
  line L137 (2.34, 29.099) -> (1.34, 29.099)
  line L138 (1.34, 29.099) -> (1.34, 28.099)
  line L139 (1.34, 31.099) -> (2.34, 31.099)
  line L140 (2.34, 31.099) -> (2.34, 32.099)
  line L141 (2.34, 32.099) -> (1.34, 32.099)
  line L142 (1.34, 32.099) -> (1.34, 31.099)
  line L143 (34.8585, 34.5556) -> (34.1514, 35.2627)
  line L144 (34.1514, 35.2627) -> (33.4443, 34.5556)
  line L145 (33.4443, 34.5556) -> (34.1514, 33.8485)
  line L146 (34.1514, 33.8485) -> (34.8585, 34.5556)
  line L147 (32.5957, 36.8184) -> (31.8886, 37.5255)
  line L148 (31.8886, 37.5255) -> (31.1815, 36.8184)
  line L149 (31.1815, 36.8184) -> (31.8886, 36.1113)
  line L150 (31.8886, 36.1113) -> (32.5957, 36.8184)
  line L151 (3.6714, 37.5255) -> (2.9643, 36.8184)
  line L152 (2.9643, 36.8184) -> (3.6714, 36.1113)
  line L153 (3.6714, 36.1113) -> (4.3785, 36.8184)
  line L154 (4.3785, 36.8184) -> (3.6714, 37.5255)
  line L155 (1.4086, 35.2627) -> (0.7015, 34.5556)
  line L156 (0.7015, 34.5556) -> (1.4086, 33.8485)
  line L157 (1.4086, 33.8485) -> (2.1157, 34.5556)
  line L158 (2.1157, 34.5556) -> (1.4086, 35.2627)
  arc A309 (7.78, 34.9567) -> (7.78, 37.1792) centre (7.78, 36.068) ccw
  arc A310 (7.78, 37.1792) -> (7.78, 34.9567) centre (7.78, 36.068) ccw
  arc A311 (7.78, 35.179) -> (7.78, 36.957) centre (7.78, 36.068) ccw
  arc A312 (7.78, 36.957) -> (7.78, 35.179) centre (7.78, 36.068) ccw
  arc A313 (7.78, 35.179) -> (7.78, 36.957) centre (7.78, 36.068) ccw
  arc A314 (7.78, 36.957) -> (7.78, 35.179) centre (7.78, 36.068) ccw
  arc A315 (7.78, 34.9567) -> (7.78, 37.1792) centre (7.78, 36.068) ccw
  arc A316 (7.78, 37.1792) -> (7.78, 34.9567) centre (7.78, 36.068) ccw
  arc A317 (27.78, 34.9567) -> (27.78, 37.1792) centre (27.78, 36.068) ccw
  arc A318 (27.78, 37.1792) -> (27.78, 34.9567) centre (27.78, 36.068) ccw
  arc A319 (27.78, 35.179) -> (27.78, 36.957) centre (27.78, 36.068) ccw
  arc A320 (27.78, 36.957) -> (27.78, 35.179) centre (27.78, 36.068) ccw
  arc A321 (27.78, 35.179) -> (27.78, 36.957) centre (27.78, 36.068) ccw
  arc A322 (27.78, 36.957) -> (27.78, 35.179) centre (27.78, 36.068) ccw
  arc A323 (27.78, 34.9567) -> (27.78, 37.1792) centre (27.78, 36.068) ccw
  arc A324 (27.78, 37.1792) -> (27.78, 34.9567) centre (27.78, 36.068) ccw
  constraints: 650 point on circle, 325 centre point, 318 end point
sketch "スケッチ4" plane through (0, 0, 0) normal (0, 0, 1) x (1, 0, 0)
  line L0 (35.56, 44.45) -> (0, 44.45) projected
  line L1 (0, 44.45) -> (0, 0) projected
  line L2 (35.56, 0) -> (35.56, 44.45) projected
  line L3 (0, 0) -> (35.56, 0) projected
  line L4 (0, 44.45) -> (35.56, 44.45)
  line L5 (35.56, 44.45) -> (35.56, 0)
  line L6 (35.56, 0) -> (0, 0)
  line L7 (0, 0) -> (0, 44.45)
  circle A0 centre (3.302, 41.148) radius 1.5
  circle A1 centre (32.258, 41.148) radius 1.5
  arc A2 (4.256, 41.148) -> (2.348, 41.148) centre (3.302, 41.148) ccw projected
  arc A3 (2.348, 41.148) -> (4.256, 41.148) centre (3.302, 41.148) ccw projected
  arc A4 (33.212, 41.148) -> (31.304, 41.148) centre (32.258, 41.148) ccw projected
  arc A5 (31.304, 41.148) -> (33.212, 41.148) centre (32.258, 41.148) ccw projected
  circle A6 centre (3.302, 41.148) radius 0.954
  circle A7 centre (32.258, 41.148) radius 0.954
  constraints: 8 end point, 4 centre point, 4 coincident, 2 concentric, 2 parallel, 1 horizontal, 1 perpendicular
extrude "押し出し3" add sketch "スケッチ4" along normal blind 3 contours L2 L3 L1 L0 | A0 | A1
sketch "スケッチ10" plane through (0, 0, 3) normal (0, 0, 1) x (1, 0, 0)
  line L0 (0, 44.45) -> (0, 0) projected
  line L1 (0, 44.45) -> (0, 0) projected
  line L2 (0, 0) -> (35.56, 0) projected
  line L3 (35.56, 0) -> (35.56, 44.45) projected
  line L4 (35.56, 44.45) -> (0, 44.45) projected
  line L5 (33.658, 7.8912) -> (33.658, 14.8808)
  line L6 (1.902, 14.8808) -> (1.902, 7.8912)
  line L7 (33.3325, 31.9891) -> (33.658, 32.0971)
  line L8 (4.702, 1.6271) -> (8.6618, 1.6271) construction
  line L9 (30.658, 6.1592) -> (24.6049, 9.654)
  line L10 (16.78, 14.1717) -> (11.1665, 17.4126)
  line L11 (11.1661, 5.3592) -> (16.78, 8.6004)
  line L12 (24.6049, 13.1181) -> (30.658, 16.6128)
  line L13 (24.3939, 5.3592) -> (18.78, 8.6004)
  line L14 (10.9551, 13.1181) -> (4.902, 16.6128)
  line L15 (4.902, 6.1592) -> (10.9551, 9.654)
  line L16 (18.78, 14.1717) -> (24.3935, 17.4126)
  line L17 (12.1665, 21.1447) -> (23.3935, 21.1447)
  arc A0 (10.9551, 9.654) -> (10.9551, 13.1181) centre (9.9551, 11.386) ccw
  arc A1 (24.6049, 13.1181) -> (24.6049, 9.654) centre (25.6049, 11.386) ccw
  arc A2 (18.78, 8.6004) -> (16.78, 8.6004) centre (17.78, 6.8683) ccw
  arc A3 (16.78, 14.1717) -> (18.78, 14.1717) centre (17.78, 15.9037) ccw
  arc A4 (4.902, 16.6128) -> (1.902, 14.8808) centre (3.902, 14.8808) ccw
  arc A5 (1.902, 7.8912) -> (4.902, 6.1592) centre (3.902, 7.8912) ccw
  arc A6 (11.1661, 5.3592) -> (12.1661, 1.6271) centre (12.1661, 3.6271) ccw
  arc A7 (23.3939, 1.6271) -> (24.3939, 5.3592) centre (23.3939, 3.6271) ccw
  arc A8 (30.658, 6.1592) -> (33.658, 7.8912) centre (31.658, 7.8912) ccw
  arc A9 (33.658, 14.8808) -> (30.658, 16.6128) centre (31.658, 14.8808) ccw
  arc A10 (24.3935, 17.4126) -> (23.3935, 21.1447) centre (23.3935, 19.1447) ccw
  arc A11 (12.1665, 21.1447) -> (11.1665, 17.4126) centre (12.1665, 19.1447) ccw
  line L18 (12.1661, 1.6271) -> (23.3939, 1.6271)
  line L19 (33.658, 29.2946) -> (33.658, 36.2841)
  line L20 (1.902, 36.2841) -> (1.902, 29.2946)
  line L21 (4.702, 23.0305) -> (8.6618, 23.0305) construction
  line L22 (30.658, 27.5625) -> (24.6049, 31.0573)
  line L23 (16.78, 35.575) -> (11.1665, 38.8159)
  line L24 (11.1661, 26.7625) -> (16.78, 30.0037)
  line L25 (24.6049, 34.5214) -> (30.658, 38.0162)
  line L26 (24.3939, 26.7625) -> (18.78, 30.0037)
  line L27 (10.9551, 34.5214) -> (4.902, 38.0162)
  line L28 (4.902, 27.5625) -> (10.9551, 31.0573)
  line L29 (18.78, 35.575) -> (24.3935, 38.8159)
  line L30 (12.1665, 42.548) -> (23.3935, 42.548)
  arc A12 (10.9551, 31.0573) -> (10.9551, 34.5214) centre (9.9551, 32.7893) ccw
  arc A13 (24.6049, 34.5214) -> (24.6049, 31.0573) centre (25.6049, 32.7893) ccw
  arc A14 (18.78, 30.0037) -> (16.78, 30.0037) centre (17.78, 28.2716) ccw
  arc A15 (16.78, 35.575) -> (18.78, 35.575) centre (17.78, 37.307) ccw
  arc A16 (4.902, 38.0162) -> (1.902, 36.2841) centre (3.902, 36.2841) ccw
  arc A17 (1.902, 29.2946) -> (4.902, 27.5625) centre (3.902, 29.2946) ccw
  arc A18 (11.1661, 26.7625) -> (12.1661, 23.0305) centre (12.1661, 25.0305) ccw
  arc A19 (23.3939, 23.0305) -> (24.3939, 26.7625) centre (23.3939, 25.0305) ccw
  arc A20 (30.658, 27.5625) -> (33.658, 29.2946) centre (31.658, 29.2946) ccw
  arc A21 (33.658, 36.2841) -> (30.658, 38.0162) centre (31.658, 36.2841) ccw
  arc A22 (24.3935, 38.8159) -> (23.3935, 42.548) centre (23.3935, 40.548) ccw
  arc A23 (12.1665, 42.548) -> (11.1665, 38.8159) centre (12.1665, 40.548) ccw
  line L31 (12.1661, 23.0305) -> (23.3939, 23.0305)
  point P0 (33.658, 1.6271)
  point P1 (33.658, 41.148)
  point P2 (1.902, 41.148)
  point P3 (30.858, 1.6271)
  point P4 (1.902, 4.4271)
  point P5 (1.902, 21.1447)
  point P6 (33.658, 21.1447)
  point P7 (33.658, 23.0305)
  point P8 (30.858, 23.0305)
  point P9 (1.902, 25.8305)
  point P10 (1.902, 42.548)
  point P11 (33.658, 42.548)
  dimension "d54" = 2
  dimension "d55" = 2
  constraints: 54 end point, 48 point on circle, 44 tangent, 24 centre point, 22 equal radius, 18 point on line, 16 parallel, 4 horizontal, 4 vertical, 2 perpendicular
  measures "d54" radius of A0
  measures "d55" radius of A12
extrude "押し出し7" cut sketch "スケッチ10" against normal blind 3 contours A8 L9 A1 L12 A9 L5 | A4 L14 A0 L15 A5 L6 | L10 A11 L17 A10 L16 A3 | L11 A2 L13 A7 L18 A6 | A20 L22 A13 L25 A21 L19 | A16 L27 A12 L28 A17 L20 | L23 A23 L30 A22 L29 A15 | L24 A14 L26 A19 L31 A18
sketch "スケッチ14" plane through (0, 0, 0) normal (0, 0, -1) x (-1, 0, 0)
  arc A0 (-12.1661, 1.6271) -> (-11.1661, 5.3592) centre (-12.1661, 3.6271) ccw projected
  line L0 (-12.1661, 1.6271) -> (-23.3939, 1.6271) projected
  arc A1 (-24.3939, 5.3592) -> (-23.3939, 1.6271) centre (-23.3939, 3.6271) ccw projected
  line L1 (-24.3939, 5.3592) -> (-18.78, 8.6004) projected
  arc A2 (-16.78, 8.6004) -> (-18.78, 8.6004) centre (-17.78, 6.8683) ccw projected
  line L2 (-16.78, 8.6004) -> (-11.1661, 5.3592) projected
  arc A3 (-18.78, 14.1717) -> (-16.78, 14.1717) centre (-17.78, 15.9037) ccw projected
  line L3 (-18.78, 14.1717) -> (-24.3935, 17.4126) projected
  arc A4 (-23.3935, 21.1447) -> (-24.3935, 17.4126) centre (-23.3935, 19.1447) ccw projected
  line L4 (-23.3935, 21.1447) -> (-12.1665, 21.1447) projected
  arc A5 (-11.1665, 17.4126) -> (-12.1665, 21.1447) centre (-12.1665, 19.1447) ccw projected
  line L5 (-11.1665, 17.4126) -> (-16.78, 14.1717) projected
  arc A6 (-33.658, 29.2946) -> (-30.658, 27.5625) centre (-31.658, 29.2946) ccw projected
  line L6 (-33.658, 29.2946) -> (-33.658, 36.2841) projected
  arc A7 (-30.658, 38.0162) -> (-33.658, 36.2841) centre (-31.658, 36.2841) ccw projected
  line L7 (-30.658, 38.0162) -> (-24.6049, 34.5214) projected
  arc A8 (-24.6049, 31.0573) -> (-24.6049, 34.5214) centre (-25.6049, 32.7893) ccw projected
  line L8 (-24.6049, 31.0573) -> (-30.658, 27.5625) projected
  arc A9 (-1.902, 14.8808) -> (-4.902, 16.6128) centre (-3.902, 14.8808) ccw projected
  line L9 (-1.902, 14.8808) -> (-1.902, 7.8912) projected
  arc A10 (-4.902, 6.1592) -> (-1.902, 7.8912) centre (-3.902, 7.8912) ccw projected
  line L10 (-4.902, 6.1592) -> (-10.9551, 9.654) projected
  arc A11 (-10.9551, 13.1181) -> (-10.9551, 9.654) centre (-9.9551, 11.386) ccw projected
  line L11 (-10.9551, 13.1181) -> (-4.902, 16.6128) projected
  arc A12 (-33.658, 7.8912) -> (-30.658, 6.1592) centre (-31.658, 7.8912) ccw projected
  line L12 (-33.658, 7.8912) -> (-33.658, 14.8808) projected
  arc A13 (-30.658, 16.6128) -> (-33.658, 14.8808) centre (-31.658, 14.8808) ccw projected
  line L13 (-30.658, 16.6128) -> (-24.6049, 13.1181) projected
  arc A14 (-24.6049, 9.654) -> (-24.6049, 13.1181) centre (-25.6049, 11.386) ccw projected
  line L14 (-24.6049, 9.654) -> (-30.658, 6.1592) projected
  arc A15 (-10.9551, 34.5214) -> (-10.9551, 31.0573) centre (-9.9551, 32.7893) ccw projected
  line L15 (-10.9551, 34.5214) -> (-4.902, 38.0162) projected
  arc A16 (-1.902, 36.2841) -> (-4.902, 38.0162) centre (-3.902, 36.2841) ccw projected
  line L16 (-1.902, 36.2841) -> (-1.902, 29.2946) projected
  arc A17 (-4.902, 27.5625) -> (-1.902, 29.2946) centre (-3.902, 29.2946) ccw projected
  line L17 (-4.902, 27.5625) -> (-10.9551, 31.0573) projected
  arc A18 (-18.78, 35.575) -> (-16.78, 35.575) centre (-17.78, 37.307) ccw projected
  line L18 (-18.78, 35.575) -> (-24.3935, 38.8159) projected
  arc A19 (-23.3935, 42.548) -> (-24.3935, 38.8159) centre (-23.3935, 40.548) ccw projected
  line L19 (-23.3935, 42.548) -> (-12.1665, 42.548) projected
  arc A20 (-11.1665, 38.8159) -> (-12.1665, 42.548) centre (-12.1665, 40.548) ccw projected
  line L20 (-11.1665, 38.8159) -> (-16.78, 35.575) projected
  arc A21 (-16.78, 30.0037) -> (-18.78, 30.0037) centre (-17.78, 28.2716) ccw projected
  line L21 (-16.78, 30.0037) -> (-11.1661, 26.7625) projected
  arc A22 (-12.1661, 23.0305) -> (-11.1661, 26.7625) centre (-12.1661, 25.0305) ccw projected
  line L22 (-12.1661, 23.0305) -> (-23.3939, 23.0305) projected
  arc A23 (-24.3939, 26.7625) -> (-23.3939, 23.0305) centre (-23.3939, 25.0305) ccw projected
  line L23 (-24.3939, 26.7625) -> (-18.78, 30.0037) projected
  line L24 (0, 44.45) -> (0, 0) projected
  line L25 (-35.56, 44.45) -> (0, 44.45) projected
  line L26 (-35.56, 0) -> (-35.56, 44.45) projected
  line L27 (0, 0) -> (-35.56, 0) projected
  line L28 (0, 44.45) -> (8, 44.45)
  line L29 (8, 44.45) -> (8, 0)
  line L30 (8, 0) -> (0, 0)
  line L31 (0, 0) -> (0, 44.45)
  dimension "d84" = 8
  constraints: 8 end point, 2 parallel, 1 horizontal, 1 perpendicular
  measures "d84" distance of L29.end L30.end
extrude "押し出し12" add sketch "スケッチ14" against normal blind 3 contours L28 L29 L30 L24
sketch "スケッチ15" plane through (0, 0, 3) normal (0, 0, 1) x (1, 0, 0)
  arc A0 (11.1661, 5.3592) -> (12.1661, 1.6271) centre (12.1661, 3.6271) ccw projected
  line L0 (11.1661, 5.3592) -> (16.78, 8.6004) projected
  arc A1 (18.78, 8.6004) -> (16.78, 8.6004) centre (17.78, 6.8683) ccw projected
  line L1 (18.78, 8.6004) -> (24.3939, 5.3592) projected
  arc A2 (23.3939, 1.6271) -> (24.3939, 5.3592) centre (23.3939, 3.6271) ccw projected
  line L2 (23.3939, 1.6271) -> (12.1661, 1.6271) projected
  arc A3 (16.78, 14.1717) -> (18.78, 14.1717) centre (17.78, 15.9037) ccw projected
  line L3 (16.78, 14.1717) -> (11.1665, 17.4126) projected
  arc A4 (12.1665, 21.1447) -> (11.1665, 17.4126) centre (12.1665, 19.1447) ccw projected
  line L4 (12.1665, 21.1447) -> (23.3935, 21.1447) projected
  arc A5 (24.3935, 17.4126) -> (23.3935, 21.1447) centre (23.3935, 19.1447) ccw projected
  line L5 (24.3935, 17.4126) -> (18.78, 14.1717) projected
  arc A6 (30.658, 27.5625) -> (33.658, 29.2946) centre (31.658, 29.2946) ccw projected
  line L6 (30.658, 27.5625) -> (24.6049, 31.0573) projected
  arc A7 (24.6049, 34.5214) -> (24.6049, 31.0573) centre (25.6049, 32.7893) ccw projected
  line L7 (24.6049, 34.5214) -> (30.658, 38.0162) projected
  arc A8 (33.658, 36.2841) -> (30.658, 38.0162) centre (31.658, 36.2841) ccw projected
  line L8 (33.658, 36.2841) -> (33.658, 29.2946) projected
  arc A9 (4.902, 16.6128) -> (1.902, 14.8808) centre (3.902, 14.8808) ccw projected
  line L9 (4.902, 16.6128) -> (10.9551, 13.1181) projected
  arc A10 (10.9551, 9.654) -> (10.9551, 13.1181) centre (9.9551, 11.386) ccw projected
  line L10 (10.9551, 9.654) -> (4.902, 6.1592) projected
  arc A11 (1.902, 7.8912) -> (4.902, 6.1592) centre (3.902, 7.8912) ccw projected
  line L11 (1.902, 7.8912) -> (1.902, 14.8808) projected
  arc A12 (30.658, 6.1592) -> (33.658, 7.8912) centre (31.658, 7.8912) ccw projected
  line L12 (30.658, 6.1592) -> (24.6049, 9.654) projected
  arc A13 (24.6049, 13.1181) -> (24.6049, 9.654) centre (25.6049, 11.386) ccw projected
  line L13 (24.6049, 13.1181) -> (30.658, 16.6128) projected
  arc A14 (33.658, 14.8808) -> (30.658, 16.6128) centre (31.658, 14.8808) ccw projected
  line L14 (33.658, 14.8808) -> (33.658, 7.8912) projected
  arc A15 (10.9551, 31.0573) -> (10.9551, 34.5214) centre (9.9551, 32.7893) ccw projected
  line L15 (10.9551, 31.0573) -> (4.902, 27.5625) projected
  arc A16 (1.902, 29.2946) -> (4.902, 27.5625) centre (3.902, 29.2946) ccw projected
  line L16 (1.902, 29.2946) -> (1.902, 36.2841) projected
  arc A17 (4.902, 38.0162) -> (1.902, 36.2841) centre (3.902, 36.2841) ccw projected
  line L17 (4.902, 38.0162) -> (10.9551, 34.5214) projected
  arc A18 (16.78, 35.575) -> (18.78, 35.575) centre (17.78, 37.307) ccw projected
  line L18 (16.78, 35.575) -> (11.1665, 38.8159) projected
  arc A19 (12.1665, 42.548) -> (11.1665, 38.8159) centre (12.1665, 40.548) ccw projected
  line L19 (12.1665, 42.548) -> (23.3935, 42.548) projected
  arc A20 (24.3935, 38.8159) -> (23.3935, 42.548) centre (23.3935, 40.548) ccw projected
  line L20 (24.3935, 38.8159) -> (18.78, 35.575) projected
  arc A21 (18.78, 30.0037) -> (16.78, 30.0037) centre (17.78, 28.2716) ccw projected
  line L21 (18.78, 30.0037) -> (24.3939, 26.7625) projected
  arc A22 (23.3939, 23.0305) -> (24.3939, 26.7625) centre (23.3939, 25.0305) ccw projected
  line L22 (23.3939, 23.0305) -> (12.1661, 23.0305) projected
  arc A23 (11.1661, 26.7625) -> (12.1661, 23.0305) centre (12.1661, 25.0305) ccw projected
  line L23 (11.1661, 26.7625) -> (16.78, 30.0037) projected
  line L24 (-8, 0) -> (35.56, 0) projected
  line L25 (35.56, 0) -> (35.56, 44.45) projected
  line L26 (35.56, 44.45) -> (-8, 44.45) projected
  line L27 (-8, 44.45) -> (-8, 0) projected
  line L28 (-8, 0) -> (-5, 0)
  line L29 (-5, 0) -> (-5, 44.45)
  line L30 (-5, 44.45) -> (-8, 44.45)
  line L31 (-8, 44.45) -> (-8, 0)
  point P0 (0, 0)
  dimension "d87" = 3
  constraints: 8 end point, 2 parallel, 1 horizontal, 1 perpendicular, 1 point on line
  measures "d87" distance of L30.end L29.end
extrude "押し出し13" add sketch "スケッチ15" along normal blind 12 contours L27 L26 L29 L24
sketch "スケッチ16" plane through (-5, 0, 3) normal (1, 0, 0) x (0, 0, -1)
  circle A0 centre (-8.5, 40.95) radius 1.6
  line L0 (-12, 0) -> (-12, 44.45) projected
  line L1 (0, 44.45) -> (-12, 44.45) projected
  circle A1 centre (-8.5, 3.5) radius 1.6
  line L2 (0, 0) -> (-12, 0) projected
  circle A2 centre (-3.5, 3.5) radius 1.6
  line L3 (0, 0) -> (0, 44.45) projected
  circle A3 centre (-3.5, 40.95) radius 1.6
  point P0 (3, 0)
  dimension "d90" = 3.2
  dimension "d91" = 3.5
  dimension "d92" = 3.5
  dimension "d93" = 3.2
  dimension "d94" = 3.5
  dimension "d95" = 3.2
  dimension "d96" = 3.5
  dimension "d97" = 3.2
  constraints: 4 centre point
  measures "d90" diameter of A0
  measures "d91" distance from line of L0 A0.centre
  measures "d92" distance from line of L1 A0.centre
  measures "d93" diameter of A1
  measures "d94" distance from line of L2 A1.centre
  measures "d95" diameter of A2
  measures "d96" distance from line of L3 A2.centre
  measures "d97" diameter of A3
extrude "押し出し14" cut sketch "スケッチ16" against normal blind 3 contours A0 | A1 | A2 | A3
chamfer "面取り3" distance 1.5 angle 45 1 edges at (-5, 22.225, 3)
sketch "スケッチ17" plane through (0, 0, 0) normal (0, 0, -1) x (-1, 0, 0)
  circle A0 centre (-32.258, 41.148) radius 0.954 projected
  line L0 (-31.1033, 43.148) -> (-29.9486, 41.148)
  line L1 (-29.9486, 41.148) -> (-31.1033, 39.148)
  line L2 (-31.1033, 39.148) -> (-33.4127, 39.148)
  line L3 (-33.4127, 39.148) -> (-34.5674, 41.148)
  line L4 (-34.5674, 41.148) -> (-33.4127, 43.148)
  line L5 (-33.4127, 43.148) -> (-31.1033, 43.148)
  circle A1 centre (-3.302, 41.148) radius 0.954 projected
  line L6 (-2.1473, 43.148) -> (-0.9926, 41.148)
  line L7 (-0.9926, 41.148) -> (-2.1473, 39.148)
  line L8 (-2.1473, 39.148) -> (-4.4567, 39.148)
  line L9 (-4.4567, 39.148) -> (-5.6114, 41.148)
  line L10 (-5.6114, 41.148) -> (-4.4567, 43.148)
  line L11 (-4.4567, 43.148) -> (-2.1473, 43.148)
  point P0 (0, 0)
  point P1 (-3.302, 41.148)
  dimension "d103" = 2
  constraints: 24 end point, 2 coincident, 26 other
  measures "d103" distance from line of L5 point (-32.258, 41.148)
extrude "押し出し15" cut sketch "スケッチ17" against normal blind 1.8
sketch "スケッチ18" plane through (0, 0, 3) normal (0, 0, 1) x (1, 0, 0)
  circle A0 centre (3.302, 41.148) radius 0.954 projected
  circle A1 centre (32.258, 41.148) radius 0.954 projected
  circle A2 centre (3.302, 41.148) radius 1.5
  circle A3 centre (32.258, 41.148) radius 1.5
  point P0 (0, 0)
  dimension "d106" = 3
  dimension "d107" = 3
  constraints: 2 centre point, 2 coincident
  measures "d106" diameter of A2
  measures "d107" diameter of A3
extrude "押し出し16" add sketch "スケッチ18" along normal blind 1.8
chamfer "面取り4" distance 1.8 angle 45 2 edges at (1.802, 41.148, 3) (30.758, 41.148, 3)
